Autodesk Fusion 360 part; units mm, degrees
(part 6 of 7)
sketch "スケッチ13" plane through (0, 0, 0) normal (0, 0, 1) x (1, 0, 0)
  arc A0 (118.5, -189.508) -> (118.5, -190.4891) centre (118.4907, -189.9985) ccw
  arc A1 (131.9907, -190.4906) -> (131.9907, -189.5094) centre (132, -190) ccw
  arc A2 (130.5532, -189.508) -> (125.4467, -189.508) centre (128, -189.9985) ccw
  spline S0 degree 5 poles (52.5, -185) (52.6382, -184.9014) (52.9088, -184.691) (53.2966, -184.3357) (53.7779, -183.7824) (54.3206, -182.9585) (54.8075, -182.0039) (55.2453, -180.9239) (55.6463, -179.7274) (56.0274, -178.4298) (56.4072, -177.0547) (56.8043, -175.6366) (57.2345, -174.223) (57.7088, -172.8764) (58.2302, -171.6789) (58.7937, -170.7262) (59.3886, -170.1082) (60, -169.8927) (60.6114, -170.1082) (61.2063, -170.7262) (61.7698, -171.6789) (62.2912, -172.8764) (62.7655, -174.223) (63.1957, -175.6366) (63.5928, -177.0547) (63.9726, -178.4298) (64.3537, -179.7274) (64.7547, -180.9239) (65.1925, -182.0039) (65.6794, -182.9585) (66.2221, -183.7824) (66.7034, -184.3357) (67.0912, -184.691) (67.3618, -184.9014) (67.5, -185) knots 0 0 0 0 0 0 0.033333 0.066667 0.1 0.133333 0.166667 0.2 0.233333 0.266667 0.3 0.333333 0.366667 0.4 0.433333 0.466667 0.5 0.533333 0.566667 0.6 0.633333 0.666667 0.7 0.733333 0.766667 0.8 0.833333 0.866667 0.9 0.933333 0.966667 1 1 1 1 1 1
  arc A3 (125.4466, -190.4891) -> (130.5533, -190.4891) centre (128, -189.9985) ccw
  spline S1 degree 5 poles (22.5, -185) (22.6382, -184.9014) (22.9088, -184.691) (23.2966, -184.3357) (23.7779, -183.7824) (24.3206, -182.9585) (24.8075, -182.0039) (25.2453, -180.9239) (25.6463, -179.7274) (26.0274, -178.4298) (26.4072, -177.0547) (26.8043, -175.6366) (27.2345, -174.223) (27.7088, -172.8764) (28.2302, -171.6789) (28.7937, -170.7262) (29.3886, -170.1082) (30, -169.8927) (30.6114, -170.1082) (31.2063, -170.7262) (31.7698, -171.6789) (32.2912, -172.8764) (32.7655, -174.223) (33.1957, -175.6366) (33.5928, -177.0547) (33.9726, -178.4298) (34.3537, -179.7274) (34.7547, -180.9239) (35.1925, -182.0039) (35.6794, -182.9585) (36.2221, -183.7824) (36.7034, -184.3357) (37.0912, -184.691) (37.3618, -184.9014) (37.5, -185) knots 0 0 0 0 0 0 0.033333 0.066667 0.1 0.133333 0.166667 0.2 0.233333 0.266667 0.3 0.333333 0.366667 0.4 0.433333 0.466667 0.5 0.533333 0.566667 0.6 0.633333 0.666667 0.7 0.733333 0.766667 0.8 0.833333 0.866667 0.9 0.933333 0.966667 1 1 1 1 1 1
  line L0 (118.4813, -190.4891) -> (125.4466, -190.4891)
  spline S2 degree 5 poles (97.5, -185) (97.6382, -184.9014) (97.9088, -184.691) (98.2966, -184.3357) (98.7779, -183.7824) (99.3206, -182.9585) (99.8075, -182.0039) (100.2453, -180.9239) (100.6463, -179.7274) (101.0274, -178.4298) (101.4072, -177.0547) (101.8043, -175.6366) (102.2345, -174.223) (102.7088, -172.8764) (103.2302, -171.6789) (103.7937, -170.7262) (104.3886, -170.1082) (105, -169.8927) (105.6114, -170.1082) (106.2063, -170.7262) (106.7698, -171.6789) (107.2912, -172.8764) (107.7655, -174.223) (108.1957, -175.6366) (108.5928, -177.0547) (108.9726, -178.4298) (109.3537, -179.7274) (109.7547, -180.9239) (110.1925, -182.0039) (110.6794, -182.9585) (111.2221, -183.7824) (111.7034, -184.3357) (112.0912, -184.691) (112.3618, -184.9014) (112.5, -185) knots 0 0 0 0 0 0 0.033333 0.066667 0.1 0.133333 0.166667 0.2 0.233333 0.266667 0.3 0.333333 0.366667 0.4 0.433333 0.466667 0.5 0.533333 0.566667 0.6 0.633333 0.666667 0.7 0.733333 0.766667 0.8 0.833333 0.866667 0.9 0.933333 0.966667 1 1 1 1 1 1
  spline S3 degree 5 poles (67.5, -185) (67.6382, -184.9014) (67.9088, -184.691) (68.2966, -184.3357) (68.7779, -183.7824) (69.3206, -182.9585) (69.8075, -182.0039) (70.2453, -180.9239) (70.6463, -179.7274) (71.0274, -178.4298) (71.4072, -177.0547) (71.8043, -175.6366) (72.2345, -174.223) (72.7088, -172.8764) (73.2302, -171.6789) (73.7937, -170.7262) (74.3886, -170.1082) (75, -169.8927) (75.6114, -170.1082) (76.2063, -170.7262) (76.7698, -171.6789) (77.2912, -172.8764) (77.7655, -174.223) (78.1957, -175.6366) (78.5928, -177.0547) (78.9726, -178.4298) (79.3537, -179.7274) (79.7547, -180.9239) (80.1925, -182.0039) (80.6794, -182.9585) (81.2221, -183.7824) (81.7034, -184.3357) (82.0912, -184.691) (82.3618, -184.9014) (82.5, -185) knots 0 0 0 0 0 0 0.033333 0.066667 0.1 0.133333 0.166667 0.2 0.233333 0.266667 0.3 0.333333 0.366667 0.4 0.433333 0.466667 0.5 0.533333 0.566667 0.6 0.633333 0.666667 0.7 0.733333 0.766667 0.8 0.833333 0.866667 0.9 0.933333 0.966667 1 1 1 1 1 1
  line L1 (125.4467, -189.508) -> (118.4813, -189.508)
  spline S4 degree 5 poles (7.5, -185) (7.6382, -184.9014) (7.9088, -184.691) (8.2966, -184.3357) (8.7779, -183.7824) (9.3206, -182.9585) (9.8075, -182.0039) (10.2453, -180.9239) (10.6463, -179.7274) (11.0274, -178.4298) (11.4072, -177.0547) (11.8043, -175.6366) (12.2345, -174.223) (12.7088, -172.8764) (13.2302, -171.6789) (13.7937, -170.7262) (14.3886, -170.1082) (15, -169.8927) (15.6114, -170.1082) (16.2063, -170.7262) (16.7698, -171.6789) (17.2912, -172.8764) (17.7655, -174.223) (18.1957, -175.6366) (18.5928, -177.0547) (18.9726, -178.4298) (19.3537, -179.7274) (19.7547, -180.9239) (20.1925, -182.0039) (20.6794, -182.9585) (21.2221, -183.7824) (21.7034, -184.3357) (22.0912, -184.691) (22.3618, -184.9014) (22.5, -185) knots 0 0 0 0 0 0 0.033333 0.066667 0.1 0.133333 0.166667 0.2 0.233333 0.266667 0.3 0.333333 0.366667 0.4 0.433333 0.466667 0.5 0.533333 0.566667 0.6 0.633333 0.666667 0.7 0.733333 0.766667 0.8 0.833333 0.866667 0.9 0.933333 0.966667 1 1 1 1 1 1
  spline S5 degree 5 poles (127.5, -185) (127.6354, -184.9046) (127.9009, -184.7005) (128.2831, -184.3542) (128.7602, -183.8116) (129.3023, -182.9962) (129.7917, -182.0427) (130.2334, -180.9541) (130.6386, -179.7408) (131.0241, -178.4225) (131.4086, -177.0279) (131.811, -175.5961) (132.2468, -174.1779) (132.7264, -172.8364) (133.2504, -171.6514) (133.8109, -170.7132) (134.2795, -170.2276) (134.6377, -170.0414) (134.8788, -170) (135, -170) knots 0 0 0 0 0 0 0.066667 0.133333 0.2 0.266667 0.333333 0.4 0.466667 0.533333 0.6 0.666667 0.733333 0.8 0.866667 0.933333 1 1 1 1 1 1
  line L2 (134.0683, -170) -> (135.9317, -170)
  spline S6 degree 5 poles (82.5, -185) (82.6382, -184.9014) (82.9088, -184.691) (83.2966, -184.3357) (83.7779, -183.7824) (84.3206, -182.9585) (84.8075, -182.0039) (85.2453, -180.9239) (85.6463, -179.7274) (86.0274, -178.4298) (86.4072, -177.0547) (86.8043, -175.6366) (87.2345, -174.223) (87.7088, -172.8764) (88.2302, -171.6789) (88.7937, -170.7262) (89.3886, -170.1082) (90, -169.8927) (90.6114, -170.1082) (91.2063, -170.7262) (91.7698, -171.6789) (92.2912, -172.8764) (92.7655, -174.223) (93.1957, -175.6366) (93.5928, -177.0547) (93.9726, -178.4298) (94.3537, -179.7274) (94.7547, -180.9239) (95.1925, -182.0039) (95.6794, -182.9585) (96.2221, -183.7824) (96.7034, -184.3357) (97.0912, -184.691) (97.3618, -184.9014) (97.5, -185) knots 0 0 0 0 0 0 0.033333 0.066667 0.1 0.133333 0.166667 0.2 0.233333 0.266667 0.3 0.333333 0.366667 0.4 0.433333 0.466667 0.5 0.533333 0.566667 0.6 0.633333 0.666667 0.7 0.733333 0.766667 0.8 0.833333 0.866667 0.9 0.933333 0.966667 1 1 1 1 1 1
  line L3 (110, -197) -> (124.5, -197)
  spline S7 degree 5 poles (37.5, -185) (37.6382, -184.9014) (37.9088, -184.691) (38.2966, -184.3357) (38.7779, -183.7824) (39.3206, -182.9585) (39.8075, -182.0039) (40.2453, -180.9239) (40.6463, -179.7274) (41.0274, -178.4298) (41.4072, -177.0547) (41.8043, -175.6366) (42.2345, -174.223) (42.7088, -172.8764) (43.2302, -171.6789) (43.7937, -170.7262) (44.3886, -170.1082) (45, -169.8927) (45.6114, -170.1082) (46.2063, -170.7262) (46.7698, -171.6789) (47.2912, -172.8764) (47.7655, -174.223) (48.1957, -175.6366) (48.5928, -177.0547) (48.9726, -178.4298) (49.3537, -179.7274) (49.7547, -180.9239) (50.1925, -182.0039) (50.6794, -182.9585) (51.2221, -183.7824) (51.7034, -184.3357) (52.0912, -184.691) (52.3618, -184.9014) (52.5, -185) knots 0 0 0 0 0 0 0.033333 0.066667 0.1 0.133333 0.166667 0.2 0.233333 0.266667 0.3 0.333333 0.366667 0.4 0.433333 0.466667 0.5 0.533333 0.566667 0.6 0.633333 0.666667 0.7 0.733333 0.766667 0.8 0.833333 0.866667 0.9 0.933333 0.966667 1 1 1 1 1 1
  spline S8 degree 5 poles (112.5, -185) (112.6382, -184.9014) (112.9088, -184.691) (113.2966, -184.3357) (113.7779, -183.7824) (114.3206, -182.9585) (114.8075, -182.0039) (115.2453, -180.9239) (115.6463, -179.7274) (116.0274, -178.4298) (116.4072, -177.0547) (116.8043, -175.6366) (117.2345, -174.223) (117.7088, -172.8764) (118.2302, -171.6789) (118.7937, -170.7262) (119.3886, -170.1082) (120, -169.8927) (120.6114, -170.1082) (121.2063, -170.7262) (121.7698, -171.6789) (122.2912, -172.8764) (122.7655, -174.223) (123.1957, -175.6366) (123.5928, -177.0547) (123.9726, -178.4298) (124.3537, -179.7274) (124.7547, -180.9239) (125.1925, -182.0039) (125.6794, -182.9585) (126.2221, -183.7824) (126.7034, -184.3357) (127.0912, -184.691) (127.3618, -184.9014) (127.5, -185) knots 0 0 0 0 0 0 0.033333 0.066667 0.1 0.133333 0.166667 0.2 0.233333 0.266667 0.3 0.333333 0.366667 0.4 0.433333 0.466667 0.5 0.533333 0.566667 0.6 0.633333 0.666667 0.7 0.733333 0.766667 0.8 0.833333 0.866667 0.9 0.933333 0.966667 1 1 1 1 1 1
  spline S9 degree 5 poles (0, -170) (0.1325, -170.0761) (0.3929, -170.246) (0.7694, -170.5546) (1.2431, -171.074) (1.7875, -171.9048) (2.2852, -172.9137) (2.7396, -174.0873) (3.1589, -175.3947) (3.5556, -176.7883) (3.9444, -178.2117) (4.3411, -179.6053) (4.7604, -180.9127) (5.2148, -182.0863) (5.7125, -183.0952) (6.2569, -183.926) (6.7306, -184.4454) (7.1071, -184.754) (7.3675, -184.9239) (7.5, -185) knots 0 0 0 0 0 0 0.066667 0.133333 0.2 0.266667 0.333333 0.4 0.466667 0.533333 0.6 0.666667 0.733333 0.8 0.866667 0.933333 1 1 1 1 1 1
  spline S10 degree 5 poles (124.5, -197) (124.9971, -197) (125.9797, -196.9323) (127.4185, -196.6274) (129.2284, -195.8334) (131.112, -194.3075) (132.4303, -192.406) (133.077, -190.3015) (133.1999, -188.1805) (133.1301, -186.1742) (133.012, -184.2924) (132.951, -182.4907) (132.9863, -180.6906) (133.1364, -178.8191) (133.409, -176.8339) (133.8064, -174.7125) (134.2233, -172.8999) (134.5905, -171.4751) (134.8595, -170.4965) (135, -170) knots 0 0 0 0 0 0 0.066667 0.133333 0.2 0.266667 0.333333 0.4 0.466667 0.533333 0.6 0.666667 0.733333 0.8 0.866667 0.933333 1 1 1 1 1 1
  line L4 (121, -197) -> (128, -197)
  line L5 (132.4806, -193.234) -> (133.5194, -186.766)
  line L6 (98, -192) -> (0, -192)
  spline S11 degree 5 poles (110, -197) (109.7722, -197) (109.3246, -196.9603) (108.6773, -196.7819) (107.855, -196.3282) (106.8563, -195.5224) (105.839, -194.6251) (104.7577, -193.7777) (103.5836, -193.0784) (102.3121, -192.5594) (100.9513, -192.2172) (99.802, -192.0667) (98.9114, -192.0121) (98.3058, -192) (98, -192) knots 0 0 0 0 0 0 0.1 0.2 0.3 0.4 0.5 0.6 0.7 0.8 0.9 1 1 1 1 1 1
  line L7 (111.2071, -197) -> (108.7929, -197)
  line L8 (99.5, -192) -> (96.5, -192)
  spline S12 degree 5 poles (-124.5, -197) (-124.9971, -197) (-125.9797, -196.9323) (-127.4185, -196.6274) (-129.2284, -195.8334) (-131.112, -194.3075) (-132.4303, -192.406) (-133.077, -190.3015) (-133.1999, -188.1805) (-133.1301, -186.1742) (-133.012, -184.2924) (-132.951, -182.4907) (-132.9863, -180.6906) (-133.1364, -178.8191) (-133.409, -176.8339) (-133.8064, -174.7125) (-134.2233, -172.8999) (-134.5905, -171.4751) (-134.8595, -170.4965) (-135, -170) knots 0 0 0 0 0 0 0.066667 0.133333 0.2 0.266667 0.333333 0.4 0.466667 0.533333 0.6 0.666667 0.733333 0.8 0.866667 0.933333 1 1 1 1 1 1
  line L9 (133.9092, -173.8541) -> (136.0908, -166.1459)
  line L10 (-121, -197) -> (-128, -197)
  line L11 (-132.4806, -193.234) -> (-133.5194, -186.766)
  line L12 (-133.9092, -173.8541) -> (-136.0908, -166.1459)
  spline S13 degree 5 poles (-127.5, -185) (-127.6354, -184.9046) (-127.9009, -184.7005) (-128.2831, -184.3542) (-128.7602, -183.8116) (-129.3023, -182.9962) (-129.7917, -182.0427) (-130.2334, -180.9541) (-130.6386, -179.7408) (-131.0241, -178.4225) (-131.4086, -177.0279) (-131.811, -175.5961) (-132.2468, -174.1779) (-132.7264, -172.8364) (-133.2504, -171.6514) (-133.8109, -170.7132) (-134.2795, -170.2276) (-134.6377, -170.0414) (-134.8788, -170) (-135, -170) knots 0 0 0 0 0 0 0.066667 0.133333 0.2 0.266667 0.333333 0.4 0.466667 0.533333 0.6 0.666667 0.733333 0.8 0.866667 0.933333 1 1 1 1 1 1
  line L13 (126.275, -185.8628) -> (128.725, -184.1372)
  line L14 (-126.275, -185.8628) -> (-128.725, -184.1372)
  line L15 (-134.0683, -170) -> (-135.9317, -170)
  spline S14 degree 5 poles (-52.5, -185) (-52.6382, -184.9014) (-52.9088, -184.691) (-53.2966, -184.3357) (-53.7779, -183.7824) (-54.3206, -182.9585) (-54.8075, -182.0039) (-55.2453, -180.9239) (-55.6463, -179.7274) (-56.0274, -178.4298) (-56.4072, -177.0547) (-56.8043, -175.6366) (-57.2345, -174.223) (-57.7088, -172.8764) (-58.2302, -171.6789) (-58.7937, -170.7262) (-59.3886, -170.1082) (-60, -169.8927) (-60.6114, -170.1082) (-61.2063, -170.7262) (-61.7698, -171.6789) (-62.2912, -172.8764) (-62.7655, -174.223) (-63.1957, -175.6366) (-63.5928, -177.0547) (-63.9726, -178.4298) (-64.3537, -179.7274) (-64.7547, -180.9239) (-65.1925, -182.0039) (-65.6794, -182.9585) (-66.2221, -183.7824) (-66.7034, -184.3357) (-67.0912, -184.691) (-67.3618, -184.9014) (-67.5, -185) knots 0 0 0 0 0 0 0.033333 0.066667 0.1 0.133333 0.166667 0.2 0.233333 0.266667 0.3 0.333333 0.366667 0.4 0.433333 0.466667 0.5 0.533333 0.566667 0.6 0.633333 0.666667 0.7 0.733333 0.766667 0.8 0.833333 0.866667 0.9 0.933333 0.966667 1 1 1 1 1 1
  line L16 (50.9927, -186.0749) -> (54.0073, -183.9251)
  line L17 (65.9927, -183.9251) -> (69.0073, -186.0749)
  line L18 (-50.9927, -186.0749) -> (-54.0073, -183.9251)
  line L19 (-65.9927, -183.9251) -> (-69.0073, -186.0749)
  arc A4 (-114.5532, -190.4992) -> (-109.4466, -190.4992) centre (-111.9999, -190.0086) ccw
  spline S15 degree 5 poles (-67.5, -185) (-67.6382, -184.9014) (-67.9088, -184.691) (-68.2966, -184.3357) (-68.7779, -183.7824) (-69.3206, -182.9585) (-69.8075, -182.0039) (-70.2453, -180.9239) (-70.6463, -179.7274) (-71.0274, -178.4298) (-71.4072, -177.0547) (-71.8043, -175.6366) (-72.2345, -174.223) (-72.7088, -172.8764) (-73.2302, -171.6789) (-73.7937, -170.7262) (-74.3886, -170.1082) (-75, -169.8927) (-75.6114, -170.1082) (-76.2063, -170.7262) (-76.7698, -171.6789) (-77.2912, -172.8764) (-77.7655, -174.223) (-78.1957, -175.6366) (-78.5928, -177.0547) (-78.9726, -178.4298) (-79.3537, -179.7274) (-79.7547, -180.9239) (-80.1925, -182.0039) (-80.6794, -182.9585) (-81.2221, -183.7824) (-81.7034, -184.3357) (-82.0912, -184.691) (-82.3618, -184.9014) (-82.5, -185) knots 0 0 0 0 0 0 0.033333 0.066667 0.1 0.133333 0.166667 0.2 0.233333 0.266667 0.3 0.333333 0.366667 0.4 0.433333 0.466667 0.5 0.533333 0.566667 0.6 0.633333 0.666667 0.7 0.733333 0.766667 0.8 0.833333 0.866667 0.9 0.933333 0.966667 1 1 1 1 1 1
  line L20 (65.9927, -186.0749) -> (69.0073, -183.9251)
  line L21 (80.9927, -183.9251) -> (84.0073, -186.0749)
  line L22 (-65.9927, -186.0749) -> (-69.0073, -183.9251)
  line L23 (-80.9927, -183.9251) -> (-84.0073, -186.0749)
  arc A5 (-109.4467, -189.4992) -> (-114.5532, -189.4992) centre (-112, -189.9897) ccw
  spline S16 degree 5 poles (-22.5, -185) (-22.6382, -184.9014) (-22.9088, -184.691) (-23.2966, -184.3357) (-23.7779, -183.7824) (-24.3206, -182.9585) (-24.8075, -182.0039) (-25.2453, -180.9239) (-25.6463, -179.7274) (-26.0274, -178.4298) (-26.4072, -177.0547) (-26.8043, -175.6366) (-27.2345, -174.223) (-27.7088, -172.8764) (-28.2302, -171.6789) (-28.7937, -170.7262) (-29.3886, -170.1082) (-30, -169.8927) (-30.6114, -170.1082) (-31.2063, -170.7262) (-31.7698, -171.6789) (-32.2912, -172.8764) (-32.7655, -174.223) (-33.1957, -175.6366) (-33.5928, -177.0547) (-33.9726, -178.4298) (-34.3537, -179.7274) (-34.7547, -180.9239) (-35.1925, -182.0039) (-35.6794, -182.9585) (-36.2221, -183.7824) (-36.7034, -184.3357) (-37.0912, -184.691) (-37.3618, -184.9014) (-37.5, -185) knots 0 0 0 0 0 0 0.033333 0.066667 0.1 0.133333 0.166667 0.2 0.233333 0.266667 0.3 0.333333 0.366667 0.4 0.433333 0.466667 0.5 0.533333 0.566667 0.6 0.633333 0.666667 0.7 0.733333 0.766667 0.8 0.833333 0.866667 0.9 0.933333 0.966667 1 1 1 1 1 1
  line L24 (20.9927, -186.0749) -> (24.0073, -183.9251)
  line L25 (35.9927, -183.9251) -> (39.0073, -186.0749)
  line L26 (-20.9927, -186.0749) -> (-24.0073, -183.9251)
  line L27 (-35.9927, -183.9251) -> (-39.0073, -186.0749)
  line L28 (-110, -197) -> (-124.5, -197)
  spline S17 degree 5 poles (-112.5, -185) (-112.6382, -184.9014) (-112.9088, -184.691) (-113.2966, -184.3357) (-113.7779, -183.7824) (-114.3206, -182.9585) (-114.8075, -182.0039) (-115.2453, -180.9239) (-115.6463, -179.7274) (-116.0274, -178.4298) (-116.4072, -177.0547) (-116.8043, -175.6366) (-117.2345, -174.223) (-117.7088, -172.8764) (-118.2302, -171.6789) (-118.7937, -170.7262) (-119.3886, -170.1082) (-120, -169.8927) (-120.6114, -170.1082) (-121.2063, -170.7262) (-121.7698, -171.6789) (-122.2912, -172.8764) (-122.7655, -174.223) (-123.1957, -175.6366) (-123.5928, -177.0547) (-123.9726, -178.4298) (-124.3537, -179.7274) (-124.7547, -180.9239) (-125.1925, -182.0039) (-125.6794, -182.9585) (-126.2221, -183.7824) (-126.7034, -184.3357) (-127.0912, -184.691) (-127.3618, -184.9014) (-127.5, -185) knots 0 0 0 0 0 0 0.033333 0.066667 0.1 0.133333 0.166667 0.2 0.233333 0.266667 0.3 0.333333 0.366667 0.4 0.433333 0.466667 0.5 0.533333 0.566667 0.6 0.633333 0.666667 0.7 0.733333 0.766667 0.8 0.833333 0.866667 0.9 0.933333 0.966667 1 1 1 1 1 1
  line L29 (110.9927, -186.0749) -> (114.0073, -183.9251)
  line L30 (125.9927, -183.9251) -> (129.0073, -186.0749)
  line L31 (-110.9927, -186.0749) -> (-114.0073, -183.9251)
  line L32 (-125.9927, -183.9251) -> (-129.0073, -186.0749)
  line L33 (-111.2071, -197) -> (-108.7929, -197)
  line L34 (-99.5, -192) -> (-96.5, -192)
  spline S18 degree 5 poles (-110, -197) (-109.531, -197) (-108.6035, -196.8979) (-107.2432, -196.4388) (-105.4719, -195.335) (-103.2255, -193.665) (-101.2961, -192.5612) (-99.7118, -192.1021) (-98.5828, -192) (-98, -192) knots 0 0 0 0 0 0 0.2 0.4 0.6 0.8 1 1 1 1 1 1
  line L35 (-111.2071, -197) -> (-108.7929, -197)
  line L36 (-99.5, -192) -> (-96.5, -192)
  spline S19 degree 5 poles (-37.5, -185) (-37.6382, -184.9014) (-37.9088, -184.691) (-38.2966, -184.3357) (-38.7779, -183.7824) (-39.3206, -182.9585) (-39.8075, -182.0039) (-40.2453, -180.9239) (-40.6463, -179.7274) (-41.0274, -178.4298) (-41.4072, -177.0547) (-41.8043, -175.6366) (-42.2345, -174.223) (-42.7088, -172.8764) (-43.2302, -171.6789) (-43.7937, -170.7262) (-44.3886, -170.1082) (-45, -169.8927) (-45.6114, -170.1082) (-46.2063, -170.7262) (-46.7698, -171.6789) (-47.2912, -172.8764) (-47.7655, -174.223) (-48.1957, -175.6366) (-48.5928, -177.0547) (-48.9726, -178.4298) (-49.3537, -179.7274) (-49.7547, -180.9239) (-50.1925, -182.0039) (-50.6794, -182.9585) (-51.2221, -183.7824) (-51.7034, -184.3357) (-52.0912, -184.691) (-52.3618, -184.9014) (-52.5, -185) knots 0 0 0 0 0 0 0.033333 0.066667 0.1 0.133333 0.166667 0.2 0.233333 0.266667 0.3 0.333333 0.366667 0.4 0.433333 0.466667 0.5 0.533333 0.566667 0.6 0.633333 0.666667 0.7 0.733333 0.766667 0.8 0.833333 0.866667 0.9 0.933333 0.966667 1 1 1 1 1 1
  line L37 (35.9927, -186.0749) -> (39.0073, -183.9251)
  line L38 (50.9927, -183.9251) -> (54.0073, -186.0749)
  line L39 (-35.9927, -186.0749) -> (-39.0073, -183.9251)
  line L40 (-50.9927, -183.9251) -> (-54.0073, -186.0749)
  spline S20 degree 5 poles (0, -170) (-0.1325, -170.0761) (-0.3929, -170.246) (-0.7694, -170.5546) (-1.2431, -171.074) (-1.7875, -171.9048) (-2.2852, -172.9137) (-2.7396, -174.0873) (-3.1589, -175.3947) (-3.5556, -176.7883) (-3.9444, -178.2117) (-4.3411, -179.6053) (-4.7604, -180.9127) (-5.2148, -182.0863) (-5.7125, -183.0952) (-6.2569, -183.926) (-6.7306, -184.4454) (-7.1071, -184.754) (-7.3675, -184.9239) (-7.5, -185) knots 0 0 0 0 0 0 0.066667 0.133333 0.2 0.266667 0.333333 0.4 0.466667 0.533333 0.6 0.666667 0.733333 0.8 0.866667 0.933333 1 1 1 1 1 1
  line L41 (-1.1777, -169.3242) -> (1.1777, -170.6758)
  line L42 (6.3223, -184.3242) -> (8.6777, -185.6758)
  line L43 (1.1777, -169.3242) -> (-1.1777, -170.6758)
  line L44 (-6.3223, -184.3242) -> (-8.6777, -185.6758)
  spline S21 degree 5 poles (-7.5, -185) (-7.6382, -184.9014) (-7.9088, -184.691) (-8.2966, -184.3357) (-8.7779, -183.7824) (-9.3206, -182.9585) (-9.8075, -182.0039) (-10.2453, -180.9239) (-10.6463, -179.7274) (-11.0274, -178.4298) (-11.4072, -177.0547) (-11.8043, -175.6366) (-12.2345, -174.223) (-12.7088, -172.8764) (-13.2302, -171.6789) (-13.7937, -170.7262) (-14.3886, -170.1082) (-15, -169.8927) (-15.6114, -170.1082) (-16.2063, -170.7262) (-16.7698, -171.6789) (-17.2912, -172.8764) (-17.7655, -174.223) (-18.1957, -175.6366) (-18.5928, -177.0547) (-18.9726, -178.4298) (-19.3537, -179.7274) (-19.7547, -180.9239) (-20.1925, -182.0039) (-20.6794, -182.9585) (-21.2221, -183.7824) (-21.7034, -184.3357) (-22.0912, -184.691) (-22.3618, -184.9014) (-22.5, -185) knots 0 0 0 0 0 0 0.033333 0.066667 0.1 0.133333 0.166667 0.2 0.233333 0.266667 0.3 0.333333 0.366667 0.4 0.433333 0.466667 0.5 0.533333 0.566667 0.6 0.633333 0.666667 0.7 0.733333 0.766667 0.8 0.833333 0.866667 0.9 0.933333 0.966667 1 1 1 1 1 1
  line L45 (5.9927, -186.0749) -> (9.0073, -183.9251)
  line L46 (20.9927, -183.9251) -> (24.0073, -186.0749)
  line L47 (-5.9927, -186.0749) -> (-9.0073, -183.9251)
  line L48 (-20.9927, -183.9251) -> (-24.0073, -186.0749)
  spline S22 degree 5 poles (-82.5, -185) (-82.6382, -184.9014) (-82.9088, -184.691) (-83.2966, -184.3357) (-83.7779, -183.7824) (-84.3206, -182.9585) (-84.8075, -182.0039) (-85.2453, -180.9239) (-85.6463, -179.7274) (-86.0274, -178.4298) (-86.4072, -177.0547) (-86.8043, -175.6366) (-87.2345, -174.223) (-87.7088, -172.8764) (-88.2302, -171.6789) (-88.7937, -170.7262) (-89.3886, -170.1082) (-90, -169.8927) (-90.6114, -170.1082) (-91.2063, -170.7262) (-91.7698, -171.6789) (-92.2912, -172.8764) (-92.7655, -174.223) (-93.1957, -175.6366) (-93.5928, -177.0547) (-93.9726, -178.4298) (-94.3537, -179.7274) (-94.7547, -180.9239) (-95.1925, -182.0039) (-95.6794, -182.9585) (-96.2221, -183.7824) (-96.7034, -184.3357) (-97.0912, -184.691) (-97.3618, -184.9014) (-97.5, -185) knots 0 0 0 0 0 0 0.033333 0.066667 0.1 0.133333 0.166667 0.2 0.233333 0.266667 0.3 0.333333 0.366667 0.4 0.433333 0.466667 0.5 0.533333 0.566667 0.6 0.633333 0.666667 0.7 0.733333 0.766667 0.8 0.833333 0.866667 0.9 0.933333 0.966667 1 1 1 1 1 1
  line L49 (80.9927, -186.0749) -> (84.0073, -183.9251)
  line L50 (95.9927, -183.9251) -> (99.0073, -186.0749)
  line L51 (-80.9927, -186.0749) -> (-84.0073, -183.9251)
  line L52 (-95.9927, -183.9251) -> (-99.0073, -186.0749)
  spline S23 degree 5 poles (-97.5, -185) (-97.6382, -184.9014) (-97.9088, -184.691) (-98.2966, -184.3357) (-98.7779, -183.7824) (-99.3206, -182.9585) (-99.8075, -182.0039) (-100.2453, -180.9239) (-100.6463, -179.7274) (-101.0274, -178.4298) (-101.4072, -177.0547) (-101.8043, -175.6366) (-102.2345, -174.223) (-102.7088, -172.8764) (-103.2302, -171.6789) (-103.7937, -170.7262) (-104.3886, -170.1082) (-105, -169.8927) (-105.6114, -170.1082) (-106.2063, -170.7262) (-106.7698, -171.6789) (-107.2912, -172.8764) (-107.7655, -174.223) (-108.1957, -175.6366) (-108.5928, -177.0547) (-108.9726, -178.4298) (-109.3537, -179.7274) (-109.7547, -180.9239) (-110.1925, -182.0039) (-110.6794, -182.9585) (-111.2221, -183.7824) (-111.7034, -184.3357) (-112.0912, -184.691) (-112.3618, -184.9014) (-112.5, -185) knots 0 0 0 0 0 0 0.033333 0.066667 0.1 0.133333 0.166667 0.2 0.233333 0.266667 0.3 0.333333 0.366667 0.4 0.433333 0.466667 0.5 0.533333 0.566667 0.6 0.633333 0.666667 0.7 0.733333 0.766667 0.8 0.833333 0.866667 0.9 0.933333 0.966667 1 1 1 1 1 1
  line L53 (95.9927, -186.0749) -> (99.0073, -183.9251)
  line L54 (110.9927, -183.9251) -> (114.0073, -186.0749)
  line L55 (-95.9927, -186.0749) -> (-99.0073, -183.9251)
  line L56 (-110.9927, -183.9251) -> (-114.0073, -186.0749)
  line L57 (-98, -192) -> (0, -192)
  line L58 (130.5532, -189.508) -> (131.9907, -189.5094)
  line L59 (131.9907, -190.4906) -> (130.5533, -190.4891)
  line L60 (-114.5532, -190.4992) -> (-118.5532, -190.4992)
  line L61 (-114.5532, -189.4992) -> (-118.5532, -189.4992)
  arc A6 (-118.5532, -189.4992) -> (-118.5532, -190.4992) centre (-118.5532, -189.9992) ccw
  line L62 (-109.4466, -190.4992) -> (-107.4467, -190.4992)
  line L63 (-109.4467, -189.4992) -> (-107.4467, -189.4992)
  arc A7 (-107.4467, -190.4992) -> (-107.4467, -189.4992) centre (-107.4467, -189.9992) ccw
  point P0 (12.5, -173.5)
  point P1 (65, -181.5)
  point P2 (80, -181.5)
  point P3 (72.5, -173.5)
  point P4 (20, -181.5)
  point P5 (92.5, -173.5)
  point P6 (15, -170)
  point P7 (105, -170)
  point P8 (2.5, -173.5)
  point P9 (85, -181.5)
  point P10 (27.5, -173.5)
  point P11 (47.5, -173.5)
  point P12 (45, -170)
  point P13 (90, -170)
  point P14 (50, -181.5)
  point P15 (30, -170)
  point P16 (32.5, -173.5)
  point P17 (57.5, -173.5)
  point P18 (55, -181.5)
  point P19 (35, -181.5)
  point P20 (95, -181.5)
  point P21 (110, -181.5)
  point P22 (102.5, -173.5)
  point P23 (40, -181.5)
  point P24 (128, -189.9985)
  point P25 (42.5, -173.5)
  point P26 (132.5, -173.5)
  point P27 (70, -181.5)
  point P28 (100, -181.5)
  point P29 (87.5, -173.5)
  point P30 (5, -181.5)
  point P31 (107.5, -173.5)
  point P32 (130, -181.5)
  point P33 (77.5, -173.5)
  point P34 (75, -170)
  point P35 (25, -181.5)
  point P36 (62.5, -173.5)
  point P37 (60, -170)
  point P38 (10, -181.5)
  point P39 (17.5, -173.5)
  point P40 (120, -170)
  point P41 (115, -181.5)
  point P42 (122.5, -173.5)
  point P43 (117.5, -173.5)
  point P44 (125, -181.5)
  point P45 (133, -190)
  point P46 (133, -181)
  point P47 (105, -194)
  point P48 (-132.5, -173.5)
  point P49 (-87.5, -173.5)
  point P50 (-17.5, -173.5)
  point P51 (-85, -181.5)
  point P52 (-2.5, -173.5)
  point P53 (-90, -170)
  point P54 (-27.5, -173.5)
  point P55 (-32.5, -173.5)
  point P56 (-72.5, -173.5)
  point P57 (-30, -170)
  point P58 (-117.5, -173.5)
  point P59 (-92.5, -173.5)
  point P60 (-75, -170)
  point P61 (-133, -181)
  point P62 (-47.5, -173.5)
  point P63 (-95, -181.5)
  point P64 (-35, -181.5)
  point P65 (-107.5, -173.5)
  point P66 (-115, -181.5)
  point P67 (-80, -181.5)
  point P68 (-70, -181.5)
  point P69 (-42.5, -173.5)
  point P70 (-40, -181.5)
  point P71 (-62.5, -173.5)
  point P72 (-45, -170)
  point P73 (-50, -181.5)
  point P74 (-57.5, -173.5)
  point P75 (-105, -170)
  point P76 (-77.5, -173.5)
  point P77 (-110, -181.5)
  point P78 (-122.5, -173.5)
  point P79 (-60, -170)
  point P80 (-120, -170)
  point P81 (-20, -181.5)
  point P82 (-10, -181.5)
  point P83 (-55, -181.5)
  point P84 (-25, -181.5)
  point P85 (-5, -181.5)
  point P86 (-65, -181.5)
  point P87 (-133, -190)
  point P88 (-15, -170)
  point P89 (-125, -181.5)
  point P90 (-130, -181.5)
  point P91 (-12.5, -173.5)
  point P92 (-102.5, -173.5)
  point P93 (-100, -181.5)
  point P94 (-118.5532, -190.4992)
  point P95 (-118.5532, -189.4992)
  dimension "d43" = 5.2
  dimension "d44" = 2.6
  dimension "d60" = 1
  dimension "d63" = 4
  dimension "d64" = 4
  dimension "d66" = 0.5
  dimension "d71" = 0.5
  constraint coincident P24 A2.centre
  constraint horizontal L0
  constraint coincident A2.start A3
  constraint concentric A2 A3
  constraint coincident A0.start L1
  constraint coincident A0.end L0
  constraint coincident L0.start A0
  constraint coincident L1.end A0
  constraint midpoint S5.end L2
  constraint midpoint L3.end L4
  constraint midpoint P45 L5
  constraint midpoint L3.start L7
  constraint coincident L3 L7.start
  constraint midpoint L6.start L8
  constraint coincident L6 L8.end
  constraint midpoint S5.end L9
  constraint midpoint S5.start L13
  constraint midpoint S0.start L16
  constraint midpoint S0.end L17
  constraint midpoint S0.end L20
  constraint midpoint S3.end L21
  constraint midpoint S1.start L24
  constraint midpoint S1.end L25
  constraint midpoint S2.end L29
  constraint midpoint S5.start L30
  constraint midpoint S1.end L37
  constraint midpoint S0.start L38
  constraint midpoint S9.start L41
  constraint midpoint S4.start L42
  constraint midpoint S4.start L45
  constraint midpoint S1.start L46
  constraint midpoint S3.end L49
  constraint midpoint S2.start L50
  constraint midpoint S2.start L53
  constraint midpoint S2.end L54
  constraint horizontal L60
  constraint horizontal L61
  constraint horizontal L62
  constraint horizontal L63
  constraint tangent L62 A7
  constraint tangent L63 A7
  measures "d43" diameter of A3
  measures "d44" radius of A3
  measures "d60" distance of L60 L61
  measures "d63" distance of A4.start P94
  measures "d64" distance of A5.end P95
  measures "d66" radius of A6
  measures "d71" radius of A7
extrude "押し出し12" add sketch "スケッチ13" along normal blind 15
sketch "スケッチ14" plane through (0, 0, 15) normal (0, 0, 1) x (-1, 0, 0)
  line L0 (-118.5, 189.508) -> (-125.4467, 189.508)
  line L1 (-125.4466, 190.4891) -> (-118.5, 190.4891)
  arc A0 (-118.5, 189.508) -> (-118.5, 190.4891) centre (-118.4907, 189.9985) ccw
  line L2 (111.2071, 197) -> (110, 197)
  spline S0 degree 5 poles (110, 197) (109.531, 197) (108.6035, 196.8979) (107.2432, 196.4388) (105.4719, 195.335) (103.2255, 193.665) (101.2961, 192.5612) (99.7118, 192.1021) (98.5828, 192) (98, 192) knots 0 0 0 0 0 0 0.2 0.4 0.6 0.8 1 1 1 1 1 1
  line L3 (98, 192) -> (-98, 192)
  spline S1 degree 5 poles (-98, 192) (-98.3058, 192) (-98.9114, 192.0121) (-99.802, 192.0667) (-100.9513, 192.2172) (-102.3121, 192.5594) (-103.5836, 193.0784) (-104.7577, 193.7777) (-105.839, 194.6251) (-106.8563, 195.5224) (-107.855, 196.3282) (-108.6773, 196.7819) (-109.3246, 196.9603) (-109.7722, 197) (-110, 197) knots -1 -1 -1 -1 -1 -1 -0.9 -0.8 -0.7 -0.6 -0.5 -0.4 -0.3 -0.2 -0.1 0 0 0 0 0 0
  line L4 (-110, 197) -> (-124.5, 197)
  spline S2 degree 5 poles (-124.5, 197) (-124.9971, 197) (-125.9797, 196.9323) (-127.4185, 196.6274) (-129.2284, 195.8334) (-131.112, 194.3075) (-132.4303, 192.406) (-133.077, 190.3015) (-133.1999, 188.1805) (-133.1301, 186.1742) (-133.012, 184.2924) (-132.951, 182.4907) (-132.9863, 180.6906) (-133.1364, 178.8191) (-133.409, 176.8339) (-133.8064, 174.7125) (-134.2233, 172.8999) (-134.5905, 171.4751) (-134.8595, 170.4965) (-135, 170) knots 0 0 0 0 0 0 0.066667 0.133333 0.2 0.266667 0.333333 0.4 0.466667 0.533333 0.6 0.666667 0.733333 0.8 0.866667 0.933333 1 1 1 1 1 1
  spline S3 degree 5 poles (-135, 170) (-134.8788, 170) (-134.6377, 170.0414) (-134.2795, 170.2276) (-133.8109, 170.7132) (-133.2504, 171.6514) (-132.7264, 172.8364) (-132.2468, 174.1779) (-131.811, 175.5961) (-131.4086, 177.0279) (-131.0241, 178.4225) (-130.6386, 179.7408) (-130.2334, 180.9541) (-129.7917, 182.0427) (-129.3023, 182.9962) (-128.7602, 183.8116) (-128.2831, 184.3542) (-127.9009, 184.7005) (-127.6354, 184.9046) (-127.5, 185) knots -1 -1 -1 -1 -1 -1 -0.933333 -0.866667 -0.8 -0.733333 -0.666667 -0.6 -0.533333 -0.466667 -0.4 -0.333333 -0.266667 -0.2 -0.133333 -0.066667 0 0 0 0 0 0
  spline S4 degree 5 poles (-127.5, 185) (-127.3618, 184.9014) (-127.0912, 184.691) (-126.7034, 184.3357) (-126.2221, 183.7824) (-125.6794, 182.9585) (-125.1925, 182.0039) (-124.7547, 180.9239) (-124.3537, 179.7274) (-123.9726, 178.4298) (-123.5928, 177.0547) (-123.1957, 175.6366) (-122.7655, 174.223) (-122.2912, 172.8764) (-121.7698, 171.6789) (-121.2063, 170.7262) (-120.6114, 170.1082) (-120, 169.8927) (-119.3886, 170.1082) (-118.7937, 170.7262) (-118.2302, 171.6789) (-117.7088, 172.8764) (-117.2345, 174.223) (-116.8043, 175.6366) (-116.4072, 177.0547) (-116.0274, 178.4298) (-115.6463, 179.7274) (-115.2453, 180.9239) (-114.8075, 182.0039) (-114.3206, 182.9585) (-113.7779, 183.7824) (-113.2966, 184.3357) (-112.9088, 184.691) (-112.6382, 184.9014) (-112.5, 185) knots -1 -1 -1 -1 -1 -1 -0.966667 -0.933333 -0.9 -0.866667 -0.833333 -0.8 -0.766667 -0.733333 -0.7 -0.666667 -0.633333 -0.6 -0.566667 -0.533333 -0.5 -0.466667 -0.433333 -0.4 -0.366667 -0.333333 -0.3 -0.266667 -0.233333 -0.2 -0.166667 -0.133333 -0.1 -0.066667 -0.033333 0 0 0 0 0 0
  spline S5 degree 5 poles (-112.5, 185) (-112.3618, 184.9014) (-112.0912, 184.691) (-111.7034, 184.3357) (-111.2221, 183.7824) (-110.6794, 182.9585) (-110.1925, 182.0039) (-109.7547, 180.9239) (-109.3537, 179.7274) (-108.9726, 178.4298) (-108.5928, 177.0547) (-108.1957, 175.6366) (-107.7655, 174.223) (-107.2912, 172.8764) (-106.7698, 171.6789) (-106.2063, 170.7262) (-105.6114, 170.1082) (-105, 169.8927) (-104.3886, 170.1082) (-103.7937, 170.7262) (-103.2302, 171.6789) (-102.7088, 172.8764) (-102.2345, 174.223) (-101.8043, 175.6366) (-101.4072, 177.0547) (-101.0274, 178.4298) (-100.6463, 179.7274) (-100.2453, 180.9239) (-99.8075, 182.0039) (-99.3206, 182.9585) (-98.7779, 183.7824) (-98.2966, 184.3357) (-97.9088, 184.691) (-97.6382, 184.9014) (-97.5, 185) knots -1 -1 -1 -1 -1 -1 -0.966667 -0.933333 -0.9 -0.866667 -0.833333 -0.8 -0.766667 -0.733333 -0.7 -0.666667 -0.633333 -0.6 -0.566667 -0.533333 -0.5 -0.466667 -0.433333 -0.4 -0.366667 -0.333333 -0.3 -0.266667 -0.233333 -0.2 -0.166667 -0.133333 -0.1 -0.066667 -0.033333 0 0 0 0 0 0
  spline S6 degree 5 poles (-97.5, 185) (-97.3618, 184.9014) (-97.0912, 184.691) (-96.7034, 184.3357) (-96.2221, 183.7824) (-95.6794, 182.9585) (-95.1925, 182.0039) (-94.7547, 180.9239) (-94.3537, 179.7274) (-93.9726, 178.4298) (-93.5928, 177.0547) (-93.1957, 175.6366) (-92.7655, 174.223) (-92.2912, 172.8764) (-91.7698, 171.6789) (-91.2063, 170.7262) (-90.6114, 170.1082) (-90, 169.8927) (-89.3886, 170.1082) (-88.7937, 170.7262) (-88.2302, 171.6789) (-87.7088, 172.8764) (-87.2345, 174.223) (-86.8043, 175.6366) (-86.4072, 177.0547) (-86.0274, 178.4298) (-85.6463, 179.7274) (-85.2453, 180.9239) (-84.8075, 182.0039) (-84.3206, 182.9585) (-83.7779, 183.7824) (-83.2966, 184.3357) (-82.9088, 184.691) (-82.6382, 184.9014) (-82.5, 185) knots -1 -1 -1 -1 -1 -1 -0.966667 -0.933333 -0.9 -0.866667 -0.833333 -0.8 -0.766667 -0.733333 -0.7 -0.666667 -0.633333 -0.6 -0.566667 -0.533333 -0.5 -0.466667 -0.433333 -0.4 -0.366667 -0.333333 -0.3 -0.266667 -0.233333 -0.2 -0.166667 -0.133333 -0.1 -0.066667 -0.033333 0 0 0 0 0 0
  spline S7 degree 5 poles (-82.5, 185) (-82.3618, 184.9014) (-82.0912, 184.691) (-81.7034, 184.3357) (-81.2221, 183.7824) (-80.6794, 182.9585) (-80.1925, 182.0039) (-79.7547, 180.9239) (-79.3537, 179.7274) (-78.9726, 178.4298) (-78.5928, 177.0547) (-78.1957, 175.6366) (-77.7655, 174.223) (-77.2912, 172.8764) (-76.7698, 171.6789) (-76.2063, 170.7262) (-75.6114, 170.1082) (-75, 169.8927) (-74.3886, 170.1082) (-73.7937, 170.7262) (-73.2302, 171.6789) (-72.7088, 172.8764) (-72.2345, 174.223) (-71.8043, 175.6366) (-71.4072, 177.0547) (-71.0274, 178.4298) (-70.6463, 179.7274) (-70.2453, 180.9239) (-69.8075, 182.0039) (-69.3206, 182.9585) (-68.7779, 183.7824) (-68.2966, 184.3357) (-67.9088, 184.691) (-67.6382, 184.9014) (-67.5, 185) knots -1 -1 -1 -1 -1 -1 -0.966667 -0.933333 -0.9 -0.866667 -0.833333 -0.8 -0.766667 -0.733333 -0.7 -0.666667 -0.633333 -0.6 -0.566667 -0.533333 -0.5 -0.466667 -0.433333 -0.4 -0.366667 -0.333333 -0.3 -0.266667 -0.233333 -0.2 -0.166667 -0.133333 -0.1 -0.066667 -0.033333 0 0 0 0 0 0
  spline S8 degree 5 poles (-67.5, 185) (-67.3618, 184.9014) (-67.0912, 184.691) (-66.7034, 184.3357) (-66.2221, 183.7824) (-65.6794, 182.9585) (-65.1925, 182.0039) (-64.7547, 180.9239) (-64.3537, 179.7274) (-63.9726, 178.4298) (-63.5928, 177.0547) (-63.1957, 175.6366) (-62.7655, 174.223) (-62.2912, 172.8764) (-61.7698, 171.6789) (-61.2063, 170.7262) (-60.6114, 170.1082) (-60, 169.8927) (-59.3886, 170.1082) (-58.7937, 170.7262) (-58.2302, 171.6789) (-57.7088, 172.8764) (-57.2345, 174.223) (-56.8043, 175.6366) (-56.4072, 177.0547) (-56.0274, 178.4298) (-55.6463, 179.7274) (-55.2453, 180.9239) (-54.8075, 182.0039) (-54.3206, 182.9585) (-53.7779, 183.7824) (-53.2966, 184.3357) (-52.9088, 184.691) (-52.6382, 184.9014) (-52.5, 185) knots -1 -1 -1 -1 -1 -1 -0.966667 -0.933333 -0.9 -0.866667 -0.833333 -0.8 -0.766667 -0.733333 -0.7 -0.666667 -0.633333 -0.6 -0.566667 -0.533333 -0.5 -0.466667 -0.433333 -0.4 -0.366667 -0.333333 -0.3 -0.266667 -0.233333 -0.2 -0.166667 -0.133333 -0.1 -0.066667 -0.033333 0 0 0 0 0 0
  spline S9 degree 5 poles (-52.5, 185) (-52.3618, 184.9014) (-52.0912, 184.691) (-51.7034, 184.3357) (-51.2221, 183.7824) (-50.6794, 182.9585) (-50.1925, 182.0039) (-49.7547, 180.9239) (-49.3537, 179.7274) (-48.9726, 178.4298) (-48.5928, 177.0547) (-48.1957, 175.6366) (-47.7655, 174.223) (-47.2912, 172.8764) (-46.7698, 171.6789) (-46.2063, 170.7262) (-45.6114, 170.1082) (-45, 169.8927) (-44.3886, 170.1082) (-43.7937, 170.7262) (-43.2302, 171.6789) (-42.7088, 172.8764) (-42.2345, 174.223) (-41.8043, 175.6366) (-41.4072, 177.0547) (-41.0274, 178.4298) (-40.6463, 179.7274) (-40.2453, 180.9239) (-39.8075, 182.0039) (-39.3206, 182.9585) (-38.7779, 183.7824) (-38.2966, 184.3357) (-37.9088, 184.691) (-37.6382, 184.9014) (-37.5, 185) knots -1 -1 -1 -1 -1 -1 -0.966667 -0.933333 -0.9 -0.866667 -0.833333 -0.8 -0.766667 -0.733333 -0.7 -0.666667 -0.633333 -0.6 -0.566667 -0.533333 -0.5 -0.466667 -0.433333 -0.4 -0.366667 -0.333333 -0.3 -0.266667 -0.233333 -0.2 -0.166667 -0.133333 -0.1 -0.066667 -0.033333 0 0 0 0 0 0
  spline S10 degree 5 poles (-37.5, 185) (-37.3618, 184.9014) (-37.0912, 184.691) (-36.7034, 184.3357) (-36.2221, 183.7824) (-35.6794, 182.9585) (-35.1925, 182.0039) (-34.7547, 180.9239) (-34.3537, 179.7274) (-33.9726, 178.4298) (-33.5928, 177.0547) (-33.1957, 175.6366) (-32.7655, 174.223) (-32.2912, 172.8764) (-31.7698, 171.6789) (-31.2063, 170.7262) (-30.6114, 170.1082) (-30, 169.8927) (-29.3886, 170.1082) (-28.7937, 170.7262) (-28.2302, 171.6789) (-27.7088, 172.8764) (-27.2345, 174.223) (-26.8043, 175.6366) (-26.4072, 177.0547) (-26.0274, 178.4298) (-25.6463, 179.7274) (-25.2453, 180.9239) (-24.8075, 182.0039) (-24.3206, 182.9585) (-23.7779, 183.7824) (-23.2966, 184.3357) (-22.9088, 184.691) (-22.6382, 184.9014) (-22.5, 185) knots -1 -1 -1 -1 -1 -1 -0.966667 -0.933333 -0.9 -0.866667 -0.833333 -0.8 -0.766667 -0.733333 -0.7 -0.666667 -0.633333 -0.6 -0.566667 -0.533333 -0.5 -0.466667 -0.433333 -0.4 -0.366667 -0.333333 -0.3 -0.266667 -0.233333 -0.2 -0.166667 -0.133333 -0.1 -0.066667 -0.033333 0 0 0 0 0 0
  spline S11 degree 5 poles (-22.5, 185) (-22.3618, 184.9014) (-22.0912, 184.691) (-21.7034, 184.3357) (-21.2221, 183.7824) (-20.6794, 182.9585) (-20.1925, 182.0039) (-19.7547, 180.9239) (-19.3537, 179.7274) (-18.9726, 178.4298) (-18.5928, 177.0547) (-18.1957, 175.6366) (-17.7655, 174.223) (-17.2912, 172.8764) (-16.7698, 171.6789) (-16.2063, 170.7262) (-15.6114, 170.1082) (-15, 169.8927) (-14.3886, 170.1082) (-13.7937, 170.7262) (-13.2302, 171.6789) (-12.7088, 172.8764) (-12.2345, 174.223) (-11.8043, 175.6366) (-11.4072, 177.0547) (-11.0274, 178.4298) (-10.6463, 179.7274) (-10.2453, 180.9239) (-9.8075, 182.0039) (-9.3206, 182.9585) (-8.7779, 183.7824) (-8.2966, 184.3357) (-7.9088, 184.691) (-7.6382, 184.9014) (-7.5, 185) knots -1 -1 -1 -1 -1 -1 -0.966667 -0.933333 -0.9 -0.866667 -0.833333 -0.8 -0.766667 -0.733333 -0.7 -0.666667 -0.633333 -0.6 -0.566667 -0.533333 -0.5 -0.466667 -0.433333 -0.4 -0.366667 -0.333333 -0.3 -0.266667 -0.233333 -0.2 -0.166667 -0.133333 -0.1 -0.066667 -0.033333 0 0 0 0 0 0
  spline S12 degree 5 poles (-7.5, 185) (-7.3675, 184.9239) (-7.1071, 184.754) (-6.7306, 184.4454) (-6.2569, 183.926) (-5.7125, 183.0952) (-5.2148, 182.0863) (-4.7604, 180.9127) (-4.3411, 179.6053) (-3.9444, 178.2117) (-3.5556, 176.7883) (-3.1589, 175.3947) (-2.7396, 174.0873) (-2.2852, 172.9137) (-1.7875, 171.9048) (-1.2431, 171.074) (-0.7694, 170.5546) (-0.3929, 170.246) (-0.1325, 170.0761) (0, 170) knots -1 -1 -1 -1 -1 -1 -0.933333 -0.866667 -0.8 -0.733333 -0.666667 -0.6 -0.533333 -0.466667 -0.4 -0.333333 -0.266667 -0.2 -0.133333 -0.066667 0 0 0 0 0 0
  spline S13 degree 5 poles (0, 170) (0.1325, 170.0761) (0.3929, 170.246) (0.7694, 170.5546) (1.2431, 171.074) (1.7875, 171.9048) (2.2852, 172.9137) (2.7396, 174.0873) (3.1589, 175.3947) (3.5556, 176.7883) (3.9444, 178.2117) (4.3411, 179.6053) (4.7604, 180.9127) (5.2148, 182.0863) (5.7125, 183.0952) (6.2569, 183.926) (6.7306, 184.4454) (7.1071, 184.754) (7.3675, 184.9239) (7.5, 185) knots 0 0 0 0 0 0 0.066667 0.133333 0.2 0.266667 0.333333 0.4 0.466667 0.533333 0.6 0.666667 0.733333 0.8 0.866667 0.933333 1 1 1 1 1 1
  spline S14 degree 5 poles (7.5, 185) (7.6382, 184.9014) (7.9088, 184.691) (8.2966, 184.3357) (8.7779, 183.7824) (9.3206, 182.9585) (9.8075, 182.0039) (10.2453, 180.9239) (10.6463, 179.7274) (11.0274, 178.4298) (11.4072, 177.0547) (11.8043, 175.6366) (12.2345, 174.223) (12.7088, 172.8764) (13.2302, 171.6789) (13.7937, 170.7262) (14.3886, 170.1082) (15, 169.8927) (15.6114, 170.1082) (16.2063, 170.7262) (16.7698, 171.6789) (17.2912, 172.8764) (17.7655, 174.223) (18.1957, 175.6366) (18.5928, 177.0547) (18.9726, 178.4298) (19.3537, 179.7274) (19.7547, 180.9239) (20.1925, 182.0039) (20.6794, 182.9585) (21.2221, 183.7824) (21.7034, 184.3357) (22.0912, 184.691) (22.3618, 184.9014) (22.5, 185) knots 0 0 0 0 0 0 0.033333 0.066667 0.1 0.133333 0.166667 0.2 0.233333 0.266667 0.3 0.333333 0.366667 0.4 0.433333 0.466667 0.5 0.533333 0.566667 0.6 0.633333 0.666667 0.7 0.733333 0.766667 0.8 0.833333 0.866667 0.9 0.933333 0.966667 1 1 1 1 1 1
  spline S15 degree 5 poles (22.5, 185) (22.6382, 184.9014) (22.9088, 184.691) (23.2966, 184.3357) (23.7779, 183.7824) (24.3206, 182.9585) (24.8075, 182.0039) (25.2453, 180.9239) (25.6463, 179.7274) (26.0274, 178.4298) (26.4072, 177.0547) (26.8043, 175.6366) (27.2345, 174.223) (27.7088, 172.8764) (28.2302, 171.6789) (28.7937, 170.7262) (29.3886, 170.1082) (30, 169.8927) (30.6114, 170.1082) (31.2063, 170.7262) (31.7698, 171.6789) (32.2912, 172.8764) (32.7655, 174.223) (33.1957, 175.6366) (33.5928, 177.0547) (33.9726, 178.4298) (34.3537, 179.7274) (34.7547, 180.9239) (35.1925, 182.0039) (35.6794, 182.9585) (36.2221, 183.7824) (36.7034, 184.3357) (37.0912, 184.691) (37.3618, 184.9014) (37.5, 185) knots 0 0 0 0 0 0 0.033333 0.066667 0.1 0.133333 0.166667 0.2 0.233333 0.266667 0.3 0.333333 0.366667 0.4 0.433333 0.466667 0.5 0.533333 0.566667 0.6 0.633333 0.666667 0.7 0.733333 0.766667 0.8 0.833333 0.866667 0.9 0.933333 0.966667 1 1 1 1 1 1
  spline S16 degree 5 poles (37.5, 185) (37.6382, 184.9014) (37.9088, 184.691) (38.2966, 184.3357) (38.7779, 183.7824) (39.3206, 182.9585) (39.8075, 182.0039) (40.2453, 180.9239) (40.6463, 179.7274) (41.0274, 178.4298) (41.4072, 177.0547) (41.8043, 175.6366) (42.2345, 174.223) (42.7088, 172.8764) (43.2302, 171.6789) (43.7937, 170.7262) (44.3886, 170.1082) (45, 169.8927) (45.6114, 170.1082) (46.2063, 170.7262) (46.7698, 171.6789) (47.2912, 172.8764) (47.7655, 174.223) (48.1957, 175.6366) (48.5928, 177.0547) (48.9726, 178.4298) (49.3537, 179.7274) (49.7547, 180.9239) (50.1925, 182.0039) (50.6794, 182.9585) (51.2221, 183.7824) (51.7034, 184.3357) (52.0912, 184.691) (52.3618, 184.9014) (52.5, 185) knots 0 0 0 0 0 0 0.033333 0.066667 0.1 0.133333 0.166667 0.2 0.233333 0.266667 0.3 0.333333 0.366667 0.4 0.433333 0.466667 0.5 0.533333 0.566667 0.6 0.633333 0.666667 0.7 0.733333 0.766667 0.8 0.833333 0.866667 0.9 0.933333 0.966667 1 1 1 1 1 1
  spline S17 degree 5 poles (52.5, 185) (52.6382, 184.9014) (52.9088, 184.691) (53.2966, 184.3357) (53.7779, 183.7824) (54.3206, 182.9585) (54.8075, 182.0039) (55.2453, 180.9239) (55.6463, 179.7274) (56.0274, 178.4298) (56.4072, 177.0547) (56.8043, 175.6366) (57.2345, 174.223) (57.7088, 172.8764) (58.2302, 171.6789) (58.7937, 170.7262) (59.3886, 170.1082) (60, 169.8927) (60.6114, 170.1082) (61.2063, 170.7262) (61.7698, 171.6789) (62.2912, 172.8764) (62.7655, 174.223) (63.1957, 175.6366) (63.5928, 177.0547) (63.9726, 178.4298) (64.3537, 179.7274) (64.7547, 180.9239) (65.1925, 182.0039) (65.6794, 182.9585) (66.2221, 183.7824) (66.7034, 184.3357) (67.0912, 184.691) (67.3618, 184.9014) (67.5, 185) knots 0 0 0 0 0 0 0.033333 0.066667 0.1 0.133333 0.166667 0.2 0.233333 0.266667 0.3 0.333333 0.366667 0.4 0.433333 0.466667 0.5 0.533333 0.566667 0.6 0.633333 0.666667 0.7 0.733333 0.766667 0.8 0.833333 0.866667 0.9 0.933333 0.966667 1 1 1 1 1 1
  spline S18 degree 5 poles (67.5, 185) (67.6382, 184.9014) (67.9088, 184.691) (68.2966, 184.3357) (68.7779, 183.7824) (69.3206, 182.9585) (69.8075, 182.0039) (70.2453, 180.9239) (70.6463, 179.7274) (71.0274, 178.4298) (71.4072, 177.0547) (71.8043, 175.6366) (72.2345, 174.223) (72.7088, 172.8764) (73.2302, 171.6789) (73.7937, 170.7262) (74.3886, 170.1082) (75, 169.8927) (75.6114, 170.1082) (76.2063, 170.7262) (76.7698, 171.6789) (77.2912, 172.8764) (77.7655, 174.223) (78.1957, 175.6366) (78.5928, 177.0547) (78.9726, 178.4298) (79.3537, 179.7274) (79.7547, 180.9239) (80.1925, 182.0039) (80.6794, 182.9585) (81.2221, 183.7824) (81.7034, 184.3357) (82.0912, 184.691) (82.3618, 184.9014) (82.5, 185) knots 0 0 0 0 0 0 0.033333 0.066667 0.1 0.133333 0.166667 0.2 0.233333 0.266667 0.3 0.333333 0.366667 0.4 0.433333 0.466667 0.5 0.533333 0.566667 0.6 0.633333 0.666667 0.7 0.733333 0.766667 0.8 0.833333 0.866667 0.9 0.933333 0.966667 1 1 1 1 1 1
  spline S19 degree 5 poles (82.5, 185) (82.6382, 184.9014) (82.9088, 184.691) (83.2966, 184.3357) (83.7779, 183.7824) (84.3206, 182.9585) (84.8075, 182.0039) (85.2453, 180.9239) (85.6463, 179.7274) (86.0274, 178.4298) (86.4072, 177.0547) (86.8043, 175.6366) (87.2345, 174.223) (87.7088, 172.8764) (88.2302, 171.6789) (88.7937, 170.7262) (89.3886, 170.1082) (90, 169.8927) (90.6114, 170.1082) (91.2063, 170.7262) (91.7698, 171.6789) (92.2912, 172.8764) (92.7655, 174.223) (93.1957, 175.6366) (93.5928, 177.0547) (93.9726, 178.4298) (94.3537, 179.7274) (94.7547, 180.9239) (95.1925, 182.0039) (95.6794, 182.9585) (96.2221, 183.7824) (96.7034, 184.3357) (97.0912, 184.691) (97.3618, 184.9014) (97.5, 185) knots 0 0 0 0 0 0 0.033333 0.066667 0.1 0.133333 0.166667 0.2 0.233333 0.266667 0.3 0.333333 0.366667 0.4 0.433333 0.466667 0.5 0.533333 0.566667 0.6 0.633333 0.666667 0.7 0.733333 0.766667 0.8 0.833333 0.866667 0.9 0.933333 0.966667 1 1 1 1 1 1
  spline S20 degree 5 poles (97.5, 185) (97.6382, 184.9014) (97.9088, 184.691) (98.2966, 184.3357) (98.7779, 183.7824) (99.3206, 182.9585) (99.8075, 182.0039) (100.2453, 180.9239) (100.6463, 179.7274) (101.0274, 178.4298) (101.4072, 177.0547) (101.8043, 175.6366) (102.2345, 174.223) (102.7088, 172.8764) (103.2302, 171.6789) (103.7937, 170.7262) (104.3886, 170.1082) (105, 169.8927) (105.6114, 170.1082) (106.2063, 170.7262) (106.7698, 171.6789) (107.2912, 172.8764) (107.7655, 174.223) (108.1957, 175.6366) (108.5928, 177.0547) (108.9726, 178.4298) (109.3537, 179.7274) (109.7547, 180.9239) (110.1925, 182.0039) (110.6794, 182.9585) (111.2221, 183.7824) (111.7034, 184.3357) (112.0912, 184.691) (112.3618, 184.9014) (112.5, 185) knots 0 0 0 0 0 0 0.033333 0.066667 0.1 0.133333 0.166667 0.2 0.233333 0.266667 0.3 0.333333 0.366667 0.4 0.433333 0.466667 0.5 0.533333 0.566667 0.6 0.633333 0.666667 0.7 0.733333 0.766667 0.8 0.833333 0.866667 0.9 0.933333 0.966667 1 1 1 1 1 1
  spline S21 degree 5 poles (112.5, 185) (112.6382, 184.9014) (112.9088, 184.691) (113.2966, 184.3357) (113.7779, 183.7824) (114.3206, 182.9585) (114.8075, 182.0039) (115.2453, 180.9239) (115.6463, 179.7274) (116.0274, 178.4298) (116.4072, 177.0547) (116.8043, 175.6366) (117.2345, 174.223) (117.7088, 172.8764) (118.2302, 171.6789) (118.7937, 170.7262) (119.3886, 170.1082) (120, 169.8927) (120.6114, 170.1082) (121.2063, 170.7262) (121.7698, 171.6789) (122.2912, 172.8764) (122.7655, 174.223) (123.1957, 175.6366) (123.5928, 177.0547) (123.9726, 178.4298) (124.3537, 179.7274) (124.7547, 180.9239) (125.1925, 182.0039) (125.6794, 182.9585) (126.2221, 183.7824) (126.7034, 184.3357) (127.0912, 184.691) (127.3618, 184.9014) (127.5, 185) knots 0 0 0 0 0 0 0.033333 0.066667 0.1 0.133333 0.166667 0.2 0.233333 0.266667 0.3 0.333333 0.366667 0.4 0.433333 0.466667 0.5 0.533333 0.566667 0.6 0.633333 0.666667 0.7 0.733333 0.766667 0.8 0.833333 0.866667 0.9 0.933333 0.966667 1 1 1 1 1 1
  spline S22 degree 5 poles (127.5, 185) (127.6354, 184.9046) (127.9009, 184.7005) (128.2831, 184.3542) (128.7602, 183.8116) (129.3023, 182.9962) (129.7917, 182.0427) (130.2334, 180.9541) (130.6386, 179.7408) (131.0241, 178.4225) (131.4086, 177.0279) (131.811, 175.5961) (132.2468, 174.1779) (132.7264, 172.8364) (133.2504, 171.6514) (133.8109, 170.7132) (134.2795, 170.2276) (134.6377, 170.0414) (134.8788, 170) (135, 170) knots 0 0 0 0 0 0 0.066667 0.133333 0.2 0.266667 0.333333 0.4 0.466667 0.533333 0.6 0.666667 0.733333 0.8 0.866667 0.933333 1 1 1 1 1 1
  spline S23 degree 5 poles (135, 170) (134.8595, 170.4965) (134.5905, 171.4751) (134.2233, 172.8999) (133.8064, 174.7125) (133.409, 176.8339) (133.1364, 178.8191) (132.9863, 180.6906) (132.951, 182.4907) (133.012, 184.2924) (133.1301, 186.1742) (133.1999, 188.1805) (133.077, 190.3015) (132.4303, 192.406) (131.112, 194.3075) (129.2284, 195.8334) (127.4185, 196.6274) (125.9797, 196.9323) (124.9971, 197) (124.5, 197) knots -1 -1 -1 -1 -1 -1 -0.933333 -0.866667 -0.8 -0.733333 -0.666667 -0.6 -0.533333 -0.466667 -0.4 -0.333333 -0.266667 -0.2 -0.133333 -0.066667 0 0 0 0 0 0
  line L5 (124.5, 197) -> (111.2071, 197)
  spline S24 degree 3 poles (-105, 172.6931) (-104.5881, 173.5183) (-104.1514, 174.7828) (-103.7668, 176.0817) (-103.2129, 177.9522) (-102.737, 179.9069) (-102.1002, 181.6203) (-101.4085, 183.4814) (-100.486, 185.1149) (-99.1355, 186.2591) (-98.9823, 186.3889) (-98.8242, 186.5122) (-98.6613, 186.6283) (-98.2742, 186.9044) (-97.8871, 187.1804) (-97.5, 187.4565) knots -0.398144 -0.398144 -0.398144 -0.398144 -0.30293 -0.30293 -0.30293 -0.165823 -0.165823 -0.165823 -0.016893 -0.016893 -0.016893 0 0 0 0.056001 0.056001 0.056001 0.056001